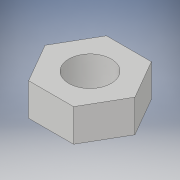
# Autodesk Inventor part: M3_Nut
Saved by Autodesk Inventor 2018 (Build 220112000, 112)
## iProperties
Created: 2020-03-27
Part Number: M3_Nut
Material: Generic
Document SubType Name: Modeling
Designer: natha
Density: 1 g/cm^3
Appearance: Default
Author: natha
Autodesk Inventor part; units mm, degrees
ref_plane "YZ Plane" through (0, 0, 0) normal (1, 0, 0) x (0, 1, 0)
ref_plane "XZ Plane" through (0, 0, 0) normal (0, 1, 0) x (-1, 0, 0)
ref_plane "XY Plane" through (0, 0, 0) normal (0, 0, 1) x (1, 0, 0)
sketch "Sketch1" plane through (0, 0, 0) normal (0, 1, 0) x (-1, 0, 0)
  line L0 (-1.5877, -2.75) -> (-3.1754, 0)
  line L1 (-3.1754, 0) -> (-1.5877, 2.75)
  line L2 (-1.5877, 2.75) -> (1.5877, 2.75)
  line L3 (1.5877, 2.75) -> (3.1754, 0)
  line L4 (3.1754, 0) -> (1.5877, -2.75)
  line L5 (1.5877, -2.75) -> (-1.5877, -2.75)
  circle A0 centre (0, 0) radius 1.5
  dimension "d0" = 5.5
  dimension "d1" = 3
  constraints: 12 end point, 1 centre point, 1 coincident
  measures "d0" distance between parallel lines of L5 L2
  measures "d1" diameter of A0
extrude "Extrusion1" add sketch "Sketch1" along normal blind 2.3
body "Solid1"
